Autodesk Fusion 360 part; units mm, degrees
(part 3 of 3)
  line L303 (-240.65, 63.65) -> (-240.65, 50.65)
  arc A300 (-193.525, 31.1) -> (-193.025, 31.6) centre (-193.525, 31.6) ccw
  line L304 (-193.525, 31.1) -> (-206.525, 31.1)
  arc A301 (-207.025, 31.6) -> (-206.525, 31.1) centre (-206.525, 31.6) ccw
  line L305 (-207.025, 31.6) -> (-207.025, 44.6)
  arc A302 (-206.525, 45.1) -> (-207.025, 44.6) centre (-206.525, 44.6) ccw
  line L306 (-206.525, 45.1) -> (-193.525, 45.1)
  arc A303 (-193.025, 44.6) -> (-193.525, 45.1) centre (-193.525, 44.6) ccw
  line L307 (-193.025, 44.6) -> (-193.025, 31.6)
  arc A304 (-117.325, 31.1) -> (-116.825, 31.6) centre (-117.325, 31.6) ccw
  line L308 (-117.325, 31.1) -> (-130.325, 31.1)
  arc A305 (-130.825, 31.6) -> (-130.325, 31.1) centre (-130.325, 31.6) ccw
  line L309 (-130.825, 31.6) -> (-130.825, 44.6)
  arc A306 (-130.325, 45.1) -> (-130.825, 44.6) centre (-130.325, 44.6) ccw
  line L310 (-130.325, 45.1) -> (-117.325, 45.1)
  arc A307 (-116.825, 44.6) -> (-117.325, 45.1) centre (-117.325, 44.6) ccw
  line L311 (-116.825, 44.6) -> (-116.825, 31.6)
  arc A308 (-212.5752, 7.287) -> (-212.0752, 7.787) centre (-212.5752, 7.787) ccw
  line L312 (-212.5752, 7.287) -> (-225.5752, 7.287)
  arc A309 (-226.0752, 7.787) -> (-225.5752, 7.287) centre (-225.5752, 7.787) ccw
  line L313 (-226.0752, 7.787) -> (-226.0752, 20.787)
  arc A310 (-225.5752, 21.287) -> (-226.0752, 20.787) centre (-225.5752, 20.787) ccw
  line L314 (-225.5752, 21.287) -> (-212.5752, 21.287)
  arc A311 (-212.0752, 20.787) -> (-212.5752, 21.287) centre (-212.5752, 20.787) ccw
  line L315 (-212.0752, 20.787) -> (-212.0752, 7.787)
  arc A312 (-53.0313, 107.3) -> (-52.5312, 107.8) centre (-53.0313, 107.8) ccw
  line L316 (-53.0313, 107.3) -> (-66.0312, 107.3)
  arc A313 (-66.5312, 107.8) -> (-66.0312, 107.3) centre (-66.0312, 107.8) ccw
  line L317 (-66.5312, 107.8) -> (-66.5313, 120.8)
  arc A314 (-66.0313, 121.3) -> (-66.5313, 120.8) centre (-66.0312, 120.8) ccw
  line L318 (-66.0312, 121.3) -> (-53.0312, 121.3)
  arc A315 (-52.5313, 120.8) -> (-53.0313, 121.3) centre (-53.0312, 120.8) ccw
  line L319 (-52.5313, 120.8) -> (-52.5312, 107.8)
  arc A316 (-150.6625, 69.2) -> (-150.1625, 69.7) centre (-150.6625, 69.7) ccw
  line L320 (-150.6625, 69.2) -> (-163.6625, 69.2)
  arc A317 (-164.1625, 69.7) -> (-163.6625, 69.2) centre (-163.6625, 69.7) ccw
  line L321 (-164.1625, 69.7) -> (-164.1625, 82.7)
  arc A318 (-163.6625, 83.2) -> (-164.1625, 82.7) centre (-163.6625, 82.7) ccw
  line L322 (-163.6625, 83.2) -> (-150.6625, 83.2)
  arc A319 (-150.1625, 82.7) -> (-150.6625, 83.2) centre (-150.6625, 82.7) ccw
  line L323 (-150.1625, 82.7) -> (-150.1625, 69.7)
  arc A320 (-124.4688, 107.3) -> (-123.9688, 107.8) centre (-124.4688, 107.8) ccw
  line L324 (-124.4688, 107.3) -> (-137.4688, 107.3)
  arc A321 (-137.9688, 107.8) -> (-137.4688, 107.3) centre (-137.4688, 107.8) ccw
  line L325 (-137.9688, 107.8) -> (-137.9688, 120.8)
  arc A322 (-137.4688, 121.3) -> (-137.9688, 120.8) centre (-137.4687, 120.8) ccw
  line L326 (-137.4688, 121.3) -> (-124.4688, 121.3)
  arc A323 (-123.9688, 120.8) -> (-124.4688, 121.3) centre (-124.4688, 120.8) ccw
  line L327 (-123.9688, 120.8) -> (-123.9688, 107.8)
  arc A324 (-184.0001, 7.287) -> (-183.5001, 7.787) centre (-184.0001, 7.787) ccw
  line L328 (-184.0001, 7.287) -> (-197.0001, 7.287)
  arc A325 (-197.5001, 7.787) -> (-197.0001, 7.287) centre (-197.0001, 7.787) ccw
  line L329 (-197.5001, 7.787) -> (-197.5001, 20.787)
  arc A326 (-197.0001, 21.287) -> (-197.5001, 20.787) centre (-197.0001, 20.787) ccw
  line L330 (-197.0001, 21.287) -> (-184.0001, 21.287)
  arc A327 (-183.5001, 20.787) -> (-184.0001, 21.287) centre (-184.0001, 20.787) ccw
  line L331 (-183.5001, 20.787) -> (-183.5001, 7.787)
  arc A328 (-164.95, 50.15) -> (-164.45, 50.65) centre (-164.95, 50.65) ccw
  line L332 (-164.95, 50.15) -> (-177.95, 50.15)
  arc A329 (-178.45, 50.65) -> (-177.95, 50.15) centre (-177.95, 50.65) ccw
  line L333 (-178.45, 50.65) -> (-178.45, 63.65)
  arc A330 (-177.95, 64.15) -> (-178.45, 63.65) centre (-177.95, 63.65) ccw
  line L334 (-177.95, 64.15) -> (-164.95, 64.15)
  arc A331 (-164.45, 63.65) -> (-164.95, 64.15) centre (-164.95, 63.65) ccw
  line L335 (-164.45, 63.65) -> (-164.45, 50.65)
  arc A332 (-291.1562, 107.3) -> (-290.6562, 107.8) centre (-291.1562, 107.8) ccw
  line L336 (-291.1562, 107.3) -> (-304.1562, 107.3)
  arc A333 (-304.6562, 107.8) -> (-304.1563, 107.3) centre (-304.1563, 107.8) ccw
  line L337 (-304.6562, 107.8) -> (-304.6562, 120.8)
  arc A334 (-304.1562, 121.3) -> (-304.6562, 120.8) centre (-304.1562, 120.8) ccw
  line L338 (-304.1562, 121.3) -> (-291.1562, 121.3)
  arc A335 (-290.6562, 120.8) -> (-291.1562, 121.3) centre (-291.1562, 120.8) ccw
  line L339 (-290.6562, 120.8) -> (-290.6563, 107.8)
  arc A336 (-74.4625, 69.2) -> (-73.9625, 69.7) centre (-74.4625, 69.7) ccw
  line L340 (-74.4625, 69.2) -> (-87.4625, 69.2)
  arc A337 (-87.9625, 69.7) -> (-87.4625, 69.2) centre (-87.4625, 69.7) ccw
  line L341 (-87.9625, 69.7) -> (-87.9625, 82.7)
  arc A338 (-87.4625, 83.2) -> (-87.9625, 82.7) centre (-87.4625, 82.7) ccw
  line L342 (-87.4625, 83.2) -> (-74.4625, 83.2)
  arc A339 (-73.9625, 82.7) -> (-74.4625, 83.2) centre (-74.4625, 82.7) ccw
  line L343 (-73.9625, 82.7) -> (-73.9625, 69.7)
  arc A340 (-55.4125, 69.2) -> (-54.9125, 69.7) centre (-55.4125, 69.7) ccw
  line L344 (-55.4125, 69.2) -> (-68.4125, 69.2)
  arc A341 (-68.9125, 69.7) -> (-68.4125, 69.2) centre (-68.4125, 69.7) ccw
  line L345 (-68.9125, 69.7) -> (-68.9125, 82.7)
  arc A342 (-68.4125, 83.2) -> (-68.9125, 82.7) centre (-68.4125, 82.7) ccw
  line L346 (-68.4125, 83.2) -> (-55.4125, 83.2)
  arc A343 (-54.9125, 82.7) -> (-55.4125, 83.2) centre (-55.4125, 82.7) ccw
  line L347 (-54.9125, 82.7) -> (-54.9125, 69.7)
  arc A344 (-131.6125, 69.2) -> (-131.1125, 69.7) centre (-131.6125, 69.7) ccw
  line L348 (-131.6125, 69.2) -> (-144.6125, 69.2)
  arc A345 (-145.1125, 69.7) -> (-144.6125, 69.2) centre (-144.6125, 69.7) ccw
  line L349 (-145.1125, 69.7) -> (-145.1125, 82.7)
  arc A346 (-144.6125, 83.2) -> (-145.1125, 82.7) centre (-144.6125, 82.7) ccw
  line L350 (-144.6125, 83.2) -> (-131.6125, 83.2)
  arc A347 (-131.1125, 82.7) -> (-131.6125, 83.2) centre (-131.6125, 82.7) ccw
  line L351 (-131.1125, 82.7) -> (-131.1125, 69.7)
  arc A348 (-41.125, 31.1) -> (-40.625, 31.6) centre (-41.125, 31.6) ccw
  line L352 (-41.125, 31.1) -> (-54.125, 31.1)
  arc A349 (-54.625, 31.6) -> (-54.125, 31.1) centre (-54.125, 31.6) ccw
  line L353 (-54.625, 31.6) -> (-54.625, 44.6)
  arc A350 (-54.125, 45.1) -> (-54.625, 44.6) centre (-54.125, 44.6) ccw
  line L354 (-54.125, 45.1) -> (-41.125, 45.1)
  arc A351 (-40.625, 44.6) -> (-41.125, 45.1) centre (-41.125, 44.6) ccw
  line L355 (-40.625, 44.6) -> (-40.625, 31.6)
  arc A352 (-231.625, 31.1) -> (-231.125, 31.6) centre (-231.625, 31.6) ccw
  line L356 (-231.625, 31.1) -> (-244.625, 31.1)
  arc A353 (-245.125, 31.6) -> (-244.625, 31.1) centre (-244.625, 31.6) ccw
  line L357 (-245.125, 31.6) -> (-245.125, 44.6)
  arc A354 (-244.625, 45.1) -> (-245.125, 44.6) centre (-244.625, 44.6) ccw
  line L358 (-244.625, 45.1) -> (-231.625, 45.1)
  arc A355 (-231.125, 44.6) -> (-231.625, 45.1) centre (-231.625, 44.6) ccw
  line L359 (-231.125, 44.6) -> (-231.125, 31.6)
  line L360 (11.2624, -9.975) -> (11.2624, 132.513)
  line L361 (8.7624, 135.013) -> (-315.9436, 135.013)
  line L362 (-318.4436, 132.513) -> (-318.4436, -9.975)
  line L363 (-315.9436, -12.475) -> (8.7624, -12.475)
  arc A356 (-318.4436, -9.975) -> (-315.9436, -12.475) centre (-315.9436, -9.975) ccw
  arc A357 (8.7624, -12.475) -> (11.2624, -9.975) centre (8.7624, -9.975) ccw
  arc A358 (11.2624, 132.513) -> (8.7624, 135.013) centre (8.7624, 132.513) ccw
  arc A359 (-315.9436, 135.013) -> (-318.4436, 132.513) centre (-315.9436, 132.513) ccw
  circle A360 centre (-314.9436, 131.513) radius 1.7
  circle A361 centre (7.7624, -8.975) radius 1.7
  circle A362 centre (7.7624, 131.513) radius 1.7
  circle A363 centre (-314.9436, -8.975) radius 1.7
  circle A364 centre (-297.6562, 14.287) radius 9.2
  dimension "d13" = 2
equation "d14 = 'JJMechanical Keyboard'"
